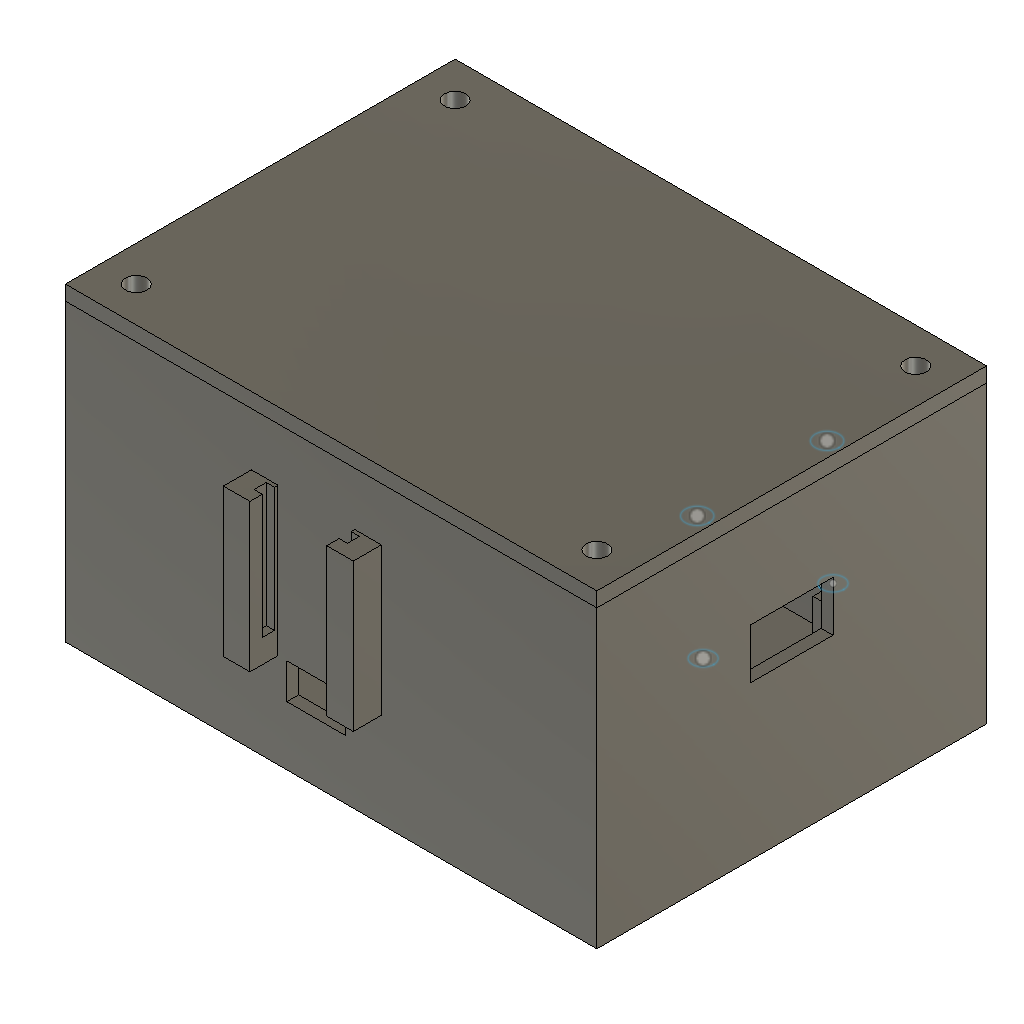
PicardSensorBoxV2 (Autodesk Fusion 360 design; units mm, degrees)
part number: 2026-09-23-13-42-49-744
part number: 2026-09-25-01-55-51-822
part number: 2026-09-25-01-55-54-357
Autodesk Fusion 360 part; units mm, degrees
ref_plane "Plan de construction1" through (0, 0, 0) normal (0, 0, 1) x (1, 0, 0) in component "Box"
sketch "Esquisse1" plane through (0, 0, 0) normal (0, 0, 1) x (1, 0, 0) in component "Box"
  line L0 (0, 0) -> (90, 0)
  line L1 (90, 0) -> (90, 66)
  line L2 (90, 66) -> (0, 66)
  line L3 (0, 66) -> (0, 0)
extrude "Extrusion1" add sketch "Esquisse1" along normal blind 2 makes body 1 in component "Box"
ref_plane "Plan de construction2" through (0, 0, 2) normal (0, 0, 1) x (1, 0, 0) in component "Box"
sketch "Esquisse2" plane through (0, 0, 2) normal (0, 0, 1) x (1, 0, 0) in component "Box"
  line L0 (0, 0) -> (90, 0)
  line L1 (90, 0) -> (90, 66)
  line L2 (90, 66) -> (0, 66)
  line L3 (0, 66) -> (0, 0)
  line L4 (2, 2) -> (88, 2)
  line L5 (88, 2) -> (88, 64)
  line L6 (88, 64) -> (2, 64)
  line L7 (2, 64) -> (2, 2)
extrude "Extrusion2" add sketch "Esquisse2" along normal blind 48 bodies 1 in component "Box"
ref_plane "Plan de construction3" through (0, 0, 2) normal (0, 0, 1) x (1, 0, 0) in component "Box"
sketch "Esquisse3" plane through (0, 0, 2) normal (0, 0, 1) x (1, 0, 0) in component "Box"
  circle A0 centre (6, 6) radius 4
  circle A1 centre (84, 6) radius 4
  circle A2 centre (6, 60) radius 4
  circle A3 centre (84, 60) radius 4
extrude "Extrusion3" add sketch "Esquisse3" along normal blind 48 bodies 1 in component "Box"
ref_plane "Plan de construction4" through (0, 0, 2) normal (0, 0, 1) x (1, 0, 0) in component "Box"
sketch "Esquisse4" plane through (0, 0, 2) normal (0, 0, 1) x (1, 0, 0) in component "Box"
  circle A0 centre (6, 6) radius 5.5
  circle A1 centre (84, 6) radius 5.5
  circle A2 centre (6, 60) radius 5.5
  circle A3 centre (84, 60) radius 5.5
extrude "Extrusion4" add sketch "Esquisse4" along normal blind 5 bodies 1 in component "Box"
ref_plane "Plan de construction5" through (0, 0, 50) normal (0, 0, 1) x (1, 0, 0) in component "Box"
sketch "Esquisse5" plane through (0, 0, 50) normal (0, 0, 1) x (1, 0, 0) in component "Box"
  circle A0 centre (6, 6) radius 1.35
  circle A1 centre (84, 6) radius 1.35
  circle A2 centre (6, 60) radius 1.35
  circle A3 centre (84, 60) radius 1.35
extrude "Extrusion5" cut sketch "Esquisse5" against normal blind 9 bodies 1 in component "Box"
ref_plane "Plan de construction6" through (0, 0, 2) normal (0, 0, 1) x (1, 0, 0) in component "Box"
sketch "Esquisse6" plane through (0, 0, 2) normal (0, 0, 1) x (1, 0, 0) in component "Box"
  line L0 (32.5, 18.5) -> (36.9, 18.5)
  line L1 (36.9, 18.5) -> (36.9, 24)
  line L2 (36.9, 24) -> (32.5, 24)
  line L3 (32.5, 24) -> (32.5, 18.5)
  line L4 (32.5, 47.5) -> (36.9, 47.5)
  line L5 (36.9, 47.5) -> (36.9, 42)
  line L6 (36.9, 42) -> (32.5, 42)
  line L7 (32.5, 42) -> (32.5, 47.5)
  line L8 (88, 18.5) -> (84.6, 18.5)
  line L9 (84.6, 18.5) -> (84.6, 24)
  line L10 (84.6, 24) -> (88, 24)
  line L11 (88, 24) -> (88, 18.5)
  line L12 (88, 47.5) -> (84.6, 47.5)
  line L13 (84.6, 47.5) -> (84.6, 42)
  line L14 (84.6, 42) -> (88, 42)
  line L15 (88, 42) -> (88, 47.5)
extrude "Extrusion6" add sketch "Esquisse6" along normal blind 26 bodies 1 in component "Box"
ref_plane "Plan de construction7" through (0, 0, 2) normal (0, 0, 1) x (1, 0, 0) in component "Box"
sketch "Esquisse7" plane through (0, 0, 2) normal (0, 0, 1) x (1, 0, 0) in component "Box"
  line L0 (29.5, 15.5) -> (36.9, 15.5)
  line L1 (36.9, 15.5) -> (36.9, 24)
  line L2 (36.9, 24) -> (29.5, 24)
  line L3 (29.5, 24) -> (29.5, 15.5)
  line L4 (29.5, 50.5) -> (36.9, 50.5)
  line L5 (36.9, 50.5) -> (36.9, 42)
  line L6 (36.9, 42) -> (29.5, 42)
  line L7 (29.5, 42) -> (29.5, 50.5)
  line L8 (88, 15.5) -> (84.6, 15.5)
  line L9 (84.6, 15.5) -> (84.6, 24)
  line L10 (84.6, 24) -> (88, 24)
  line L11 (88, 24) -> (88, 15.5)
  line L12 (88, 50.5) -> (84.6, 50.5)
  line L13 (84.6, 50.5) -> (84.6, 42)
  line L14 (84.6, 42) -> (88, 42)
  line L15 (88, 42) -> (88, 50.5)
extrude "Extrusion7" add sketch "Esquisse7" along normal blind 5 bodies 1 in component "Box"
ref_plane "Plan de construction8" through (0, 0, 28) normal (0, 0, 1) x (1, 0, 0) in component "Box"
sketch "Esquisse8" plane through (0, 0, 28) normal (0, 0, 1) x (1, 0, 0) in component "Box"
  circle A0 centre (35.5, 22) radius 1.3
  circle A1 centre (35.5, 44) radius 1.3
  circle A2 centre (86, 22) radius 1.3
  circle A3 centre (86, 44) radius 1.3
extrude "Extrusion8" add sketch "Esquisse8" along normal blind 1.4 bodies 1 in component "Box"
ref_plane "Plan de construction9" through (90, 0, 0) normal (1, 0, 0) x (0, 1, 0) in component "Box"
sketch "Esquisse9" plane through (90, 0, 0) normal (1, 0, 0) x (0, 0, -1) in component "Box"
  line L0 (-26, 26) -> (-34.5, 26)
  line L1 (-34.5, 26) -> (-34.5, 40)
  line L2 (-34.5, 40) -> (-26, 40)
  line L3 (-26, 40) -> (-26, 26)
extrude "Extrusion9" cut sketch "Esquisse9" along normal mid plane 8 bodies 1 in component "Box"
ref_plane "Plan de construction10" through (0, 0, 0) normal (1, 0, 0) x (0, 1, 0) in component "Box"
sketch "Esquisse10" plane through (0, 0, 0) normal (1, 0, 0) x (0, 0, -1) in component "Box"
  circle A0 centre (-30, 20.5) radius 8.8
extrude "Extrusion10" cut sketch "Esquisse10" along normal mid plane 8 bodies 1 in component "Box"
ref_plane "Plan de construction11" through (0, 0, 0) normal (1, 0, 0) x (0, 1, 0) in component "Box"
sketch "Esquisse11" plane through (0, 0, 0) normal (1, 0, 0) x (0, 0, -1) in component "Box"
  circle A0 centre (-30, 45.5) radius 8.8
extrude "Extrusion11" cut sketch "Esquisse11" along normal mid plane 8 bodies 1 in component "Box"
ref_plane "Plan de construction12" through (0, 0, 16) normal (0, 0, 1) x (1, 0, 0) in component "Box"
sketch "Esquisse12" plane through (0, 0, 16) normal (0, 0, 1) x (1, 0, 0) in component "Box"
  line L0 (2, 2) -> (19.1, 2)
  line L1 (19.1, 2) -> (19.1, 11.5)
  line L2 (19.1, 11.5) -> (2, 11.5)
  line L3 (2, 11.5) -> (2, 2)
  line L4 (2, 54.5) -> (19.1, 54.5)
  line L5 (19.1, 54.5) -> (19.1, 64)
  line L6 (19.1, 64) -> (2, 64)
  line L7 (2, 64) -> (2, 54.5)
extrude "Extrusion12" add sketch "Esquisse12" along normal blind 26 bodies 1 in component "Box"
ref_plane "Plan de construction13" through (0, 0, 20) normal (0, 0, 1) x (1, 0, 0) in component "Box"
sketch "Esquisse13" plane through (0, 0, 20) normal (0, 0, 1) x (1, 0, 0) in component "Box"
  line L0 (14.1, 10.1) -> (16.5, 10.1)
  line L1 (16.5, 10.1) -> (16.5, 11.5)
  line L2 (16.5, 11.5) -> (14.1, 11.5)
  line L3 (14.1, 11.5) -> (14.1, 10.1)
  line L4 (14.1, 54.5) -> (16.5, 54.5)
  line L5 (16.5, 54.5) -> (16.5, 55.9)
  line L6 (16.5, 55.9) -> (14.1, 55.9)
  line L7 (14.1, 55.9) -> (14.1, 54.5)
extrude "Extrusion13" cut sketch "Esquisse13" along normal blind 25 bodies 1 in component "Box"
ref_plane "Plan de construction14" through (0, 0, 16) normal (0, 0, 1) x (1, 0, 0) in component "Box"
sketch "Esquisse14" plane through (0, 0, 16) normal (0, 0, 1) x (1, 0, 0) in component "Box"
  line L0 (31.5, -4.75) -> (36, -4.75)
  line L1 (36, -4.75) -> (36, 0)
  line L2 (36, 0) -> (31.5, 0)
  line L3 (31.5, 0) -> (31.5, -4.75)
  line L4 (49, -4.75) -> (53.5, -4.75)
  line L5 (53.5, -4.75) -> (53.5, 0)
  line L6 (53.5, 0) -> (49, 0)
  line L7 (49, 0) -> (49, -4.75)
extrude "Extrusion14" add sketch "Esquisse14" along normal blind 25 bodies 1 in component "Box"
ref_plane "Plan de construction15" through (0, 0, 20) normal (0, 0, 1) x (1, 0, 0) in component "Box"
sketch "Esquisse15" plane through (0, 0, 20) normal (0, 0, 1) x (1, 0, 0) in component "Box"
  line L0 (34.6, -2.65) -> (36, -2.65)
  line L1 (36, -2.65) -> (36, -0.6)
  line L2 (36, -0.6) -> (34.6, -0.6)
  line L3 (34.6, -0.6) -> (34.6, -2.65)
  line L4 (49, -2.65) -> (50.4, -2.65)
  line L5 (50.4, -2.65) -> (50.4, -0.6)
  line L6 (50.4, -0.6) -> (49, -0.6)
  line L7 (49, -0.6) -> (49, -2.65)
extrude "Extrusion15" cut sketch "Esquisse15" along normal blind 24 bodies 1 in component "Box"
ref_plane "Plan de construction16" through (0, 0, 0) normal (0, 1, 0) x (0, 0, 1) in component "Box"
sketch "Esquisse16" plane through (0, 0, 0) normal (0, 1, 0) x (1, 0, 0) in component "Box"
  line L0 (37.5, -10) -> (47.5, -10)
  line L1 (47.5, -10) -> (47.5, -16)
  line L2 (47.5, -16) -> (37.5, -16)
  line L3 (37.5, -16) -> (37.5, -10)
extrude "Extrusion16" cut sketch "Esquisse16" along normal mid plane 8 bodies 1 in component "Box"
ref_plane "Plan de construction17" through (0, 0, 2) normal (0, 0, 1) x (1, 0, 0) in component "Box"
sketch "Esquisse17" plane through (0, 0, 2) normal (0, 0, 1) x (1, 0, 0) in component "Box"
  line L0 (3.5, 26.5) -> (86.5, 26.5)
  line L1 (86.5, 26.5) -> (86.5, 28)
  line L2 (86.5, 28) -> (3.5, 28)
  line L3 (3.5, 28) -> (3.5, 26.5)
  line L4 (3.5, 38) -> (86.5, 38)
  line L5 (86.5, 38) -> (86.5, 39.5)
  line L6 (86.5, 39.5) -> (3.5, 39.5)
  line L7 (3.5, 39.5) -> (3.5, 38)
  line L8 (2, 28) -> (3.5, 28)
  line L9 (3.5, 28) -> (3.5, 38)
  line L10 (3.5, 38) -> (2, 38)
  line L11 (2, 38) -> (2, 28)
  line L12 (86.5, 28) -> (88, 28)
  line L13 (88, 28) -> (88, 38)
  line L14 (88, 38) -> (86.5, 38)
  line L15 (86.5, 38) -> (86.5, 28)
extrude "Extrusion17" add sketch "Esquisse17" along normal blind 3 contours L0 L1 L2 L3 | L8 L9 L10 L11 | L12 L13 L14 L15 | L4 L5 L6 L7 bodies 1 in component "Box"
ref_plane "Plan de construction1" through (0, 0, 50) normal (0, 0, 1) x (1, 0, 0) in component "Lid"
sketch "Esquisse1 (2)" plane through (0, 0, 50) normal (0, 0, 1) x (1, 0, 0) in component "Lid"
  line L0 (0, 0) -> (90, 0)
  line L1 (90, 0) -> (90, 66)
  line L2 (90, 66) -> (0, 66)
  line L3 (0, 66) -> (0, 0)
extrude "Extrusion1'" add sketch "Esquisse1 (2)" along normal blind 2.5 separate body makes body 2 in component "Lid"
ref_plane "Plan de construction2" through (0, 0, 50) normal (0, 0, 1) x (1, 0, 0) in component "Lid"
sketch "Esquisse2 (2)" plane through (0, 0, 50) normal (0, 0, 1) x (1, 0, 0) in component "Lid"
  line L0 (2.5, 2.5) -> (87.5, 2.5)
  line L1 (87.5, 2.5) -> (87.5, 63.5)
  line L2 (87.5, 63.5) -> (2.5, 63.5)
  line L3 (2.5, 63.5) -> (2.5, 2.5)
  circle A0 centre (6, 6) radius 4.5
  circle A1 centre (84, 6) radius 4.5
  circle A2 centre (6, 60) radius 4.5
  circle A3 centre (84, 60) radius 4.5
extrude "Extrusion2'" add sketch "Esquisse2 (2)" against normal blind 3 contours L0 L1 L2 L3 A0 A1 A2 A3 bodies 2 in component "Lid"
ref_plane "Plan de construction3" through (0, 0, 52.5) normal (0, 0, 1) x (1, 0, 0) in component "Lid"
sketch "Esquisse3 (2)" plane through (0, 0, 52.5) normal (0, 0, 1) x (1, 0, 0) in component "Lid"
  circle A0 centre (6, 6) radius 1.8
  circle A1 centre (84, 6) radius 1.8
  circle A2 centre (6, 60) radius 1.8
  circle A3 centre (84, 60) radius 1.8
extrude "Extrusion18" cut sketch "Esquisse3 (2)" against normal blind 7 bodies 1 in component "Box"
extrude "Extrusion3'" cut sketch "Esquisse3 (2)" against normal blind 7 bodies 2 in component "Lid"
ref_plane "Plan de construction4" through (0, 0, 50) normal (0, 0, 1) x (1, 0, 0) in component "Lid"
sketch "Esquisse4 (2)" plane through (0, 0, 50) normal (0, 0, 1) x (1, 0, 0) in component "Lid"
  circle A0 centre (35.5, 22) radius 2
  circle A1 centre (35.5, 44) radius 2
extrude "Extrusion4'" add sketch "Esquisse4 (2)" against normal blind 20.4 bodies 2 in component "Lid"
ref_plane "Plan de construction5" through (0, 0, 50) normal (0, 0, 1) x (1, 0, 0) in component "Lid"
sketch "Esquisse5 (2)" plane through (0, 0, 50) normal (0, 0, 1) x (1, 0, 0) in component "Lid"
  circle A0 centre (85, 22) radius 2
ref_plane "Plan de construction6" through (0, 0, 29.6) normal (0, 0, 1) x (1, 0, 0) in component "Lid"
sketch "Esquisse6 (2)" plane through (0, 0, 29.6) normal (0, 0, 1) x (1, 0, 0) in component "Lid"
  circle A0 centre (86, 22) radius 1.8
loft "Lissage1" add profiles "Esquisse5 (2)", "Esquisse6 (2)" section 1 section 2 bodies 2 in component "Lid"
ref_plane "Plan de construction7" through (0, 0, 50) normal (0, 0, 1) x (1, 0, 0) in component "Lid"
sketch "Esquisse7 (2)" plane through (0, 0, 50) normal (0, 0, 1) x (1, 0, 0) in component "Lid"
  circle A0 centre (85, 44) radius 2
ref_plane "Plan de construction8" through (0, 0, 29.6) normal (0, 0, 1) x (1, 0, 0) in component "Lid"
sketch "Esquisse8 (2)" plane through (0, 0, 29.6) normal (0, 0, 1) x (1, 0, 0) in component "Lid"
  circle A0 centre (86, 44) radius 1.8
loft "Lissage2" add profiles "Esquisse7 (2)", "Esquisse8 (2)" section 1 section 2 bodies 2 in component "Lid"
component "Box" placed x (1, 0, 0) y (0, 1, 0) z (0, 0, 1) at (0, 0, 0)
component "Lid" placed x (1, 0, 0) y (0, 1, 0) z (0, 0, 1) at (0, 0, 0)
named bodies: "box", "lid"
